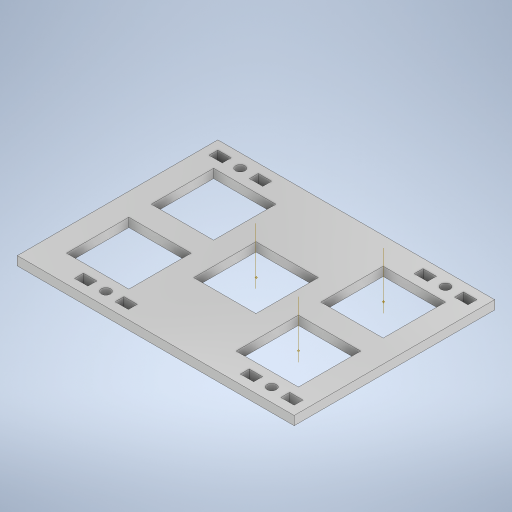
# Autodesk Inventor part: tc_base_plate
Saved by Autodesk Inventor 2024.1 (Build 281209000, 209)
## iProperties
Created: 2019-07-03
Part Number: tc_base_plate
Material: Acier inoxydable
Document SubType Name: Modeling
Designer: Thibault
Density: 8 g/cm^3
Appearance: Aluminium - Poli
Mass: 33.3223 g
Surface Area: 56.2435 cm^2
Volume: 4.16528 cm^3
tc_base_width: 62,200 mm
tc_base_support_dist: 37,050 mm
Author: Thibault
Autodesk Inventor part; units mm, degrees
ref_plane "YZ Plane" through (0, 0, 0) normal (1, 0, 0) x (0, 1, 0)
ref_plane "XZ Plane" through (0, 0, 0) normal (0, 1, 0) x (-1, 0, 0)
ref_plane "XY Plane" through (0, 0, 0) normal (0, 0, 1) x (1, 0, 0)
sketch "anchor" plane through (0, 0, 0) normal (0, 0, 1) x (1, 0, 0)
  circle A0 centre (94.2814, 48.5827) radius 0.85
  line L0 (91.2814, 49.5827) -> (87.2814, 49.5827)
  line L1 (87.2814, 49.5827) -> (87.2814, 47.5827)
  line L2 (87.2814, 47.5827) -> (91.2814, 47.5827)
  line L3 (91.2814, 47.5827) -> (91.2814, 49.5827)
  line L4 (101.2814, 49.5827) -> (97.2814, 49.5827)
  line L5 (97.2814, 49.5827) -> (97.2814, 47.5827)
  line L6 (97.2814, 47.5827) -> (101.2814, 47.5827)
  line L7 (101.2814, 47.5827) -> (101.2814, 49.5827)
  line L8 (91.2814, 49.5827) -> (97.2814, 47.5827) construction
  line L9 (97.2814, 49.5827) -> (91.2814, 47.5827) construction
  line L10 (87.2814, 51.1827) -> (101.2814, 51.1827)
  point P0 (103.5798, 50.1132)
  point P1 (94.2814, 48.5827)
  dimension "d226" = 1.7
  dimension "d230" = 4
  dimension "d231" = 2
  dimension "d237" = 4
  dimension "d245" = 1.6
  dimension "d247" = 6
  measures "d226" diameter of A0
  measures "d230" distance of L2.end L1.end
  measures "d231" distance of L1.end L0.end
  measures "d237" distance of L6.end L5.end
  measures "d245" distance between parallel lines of L0 L10
  measures "d247" distance between parallel lines of L5 L3
sketch "screw_anchor" plane through (0, 0, 0) normal (0, 0, 1) x (1, 0, 0)
  point P0 (61.1245, 15.5217)
  dimension "d155" = 14
  dimension "d156" = 19.05
  dimension "d157" = 19.05
  dimension "d158" = 19.05
  dimension "d159" = 28.575
  dimension "d160" = 19.05
  dimension "d161" = 2
  dimension "d162" = 2
  dimension "d163" = 2
  dimension "d164" = 2
  dimension "d165" = 2
  dimension "d166" = 1
  dimension "d167" = 5
  dimension "d168" = 5
  dimension "d169" = 4
sketch "Anchor (nut side)" plane through (0, 0, 0) normal (0, 0, 1) x (1, 0, 0)
  line L0 (11.1, 0) -> (9.1, 0)
  line L1 (9.1, 0) -> (9.1, -2)
  line L2 (9.1, -2) -> (9.9, -2)
  line L3 (9.9, -2) -> (9.9, -4)
  line L4 (6.2, -4) -> (6.2, -2)
  line L5 (6.2, -2) -> (7, -2)
  line L6 (7, -2) -> (7, 0)
  line L7 (7, 0) -> (5, 0)
  line L8 (2, 0) -> (2, 2)
  line L9 (2, 0) -> (3, 0) construction
  line L10 (2, 2) -> (5, 2)
  line L11 (5, 2) -> (5, 0)
  line L12 (11.1, 0) -> (11.1, 2)
  line L13 (11.1, 2) -> (14.1, 2)
  line L14 (14.1, 2) -> (14.1, 0)
  line L15 (0, 0) -> (2, 0)
  line L16 (14.1, 0) -> (16.1, 0)
  line L17 (6.2, -4) -> (7, -4)
  line L18 (9.9, -4) -> (9.1, -4)
  line L19 (7, -4) -> (7, -6.25)
  line L20 (9.1, -4) -> (9.1, -6.25)
  line L21 (7.25, -6.5) -> (8.05, -6.5)
  arc A0 (7, -6.25) -> (7.25, -6.5) centre (7.25, -6.25) ccw
  arc A1 (8.85, -6.5) -> (9.1, -6.25) centre (8.85, -6.25) ccw
  line L22 (8.05, -6.5) -> (8.85, -6.5)
  line L23 (8.05, -3.8983) -> (8.05, -9.959) construction
  point P0 (9.1321, -0.6227)
  point P1 (7, -6.5)
  point P2 (9.1, -6.5)
  dimension "d3" = 2
  dimension "d7" = 6.1
  dimension "d10" = 2
  dimension "d11" = 2
  dimension "d12" = 0.8
  dimension "d13" = 2
  dimension "d14" = 0.8
  dimension "d15" = 2.1
  dimension "d18" = 2
  dimension "d19" = 0.8
  dimension "d20" = 0.8
  dimension "d21" = 2.5
  dimension "d22" = 2.5
  dimension "d23" = 2.1
  dimension "d38" = 2
  dimension "d39" = 0.25
  dimension "d120" = 3
  measures "d3" distance of L15.start L8.start
  measures "d7" distance of L7.end L0.start
  measures "d10" distance of L0.start L0.end
  measures "d11" distance of L0.end L1.end
  measures "d12" distance of L1.end L2.end
  measures "d13" distance of L2.end L3.end
  measures "d14" distance of L4.end L5.end
  measures "d15" distance of L6.end L0.end
  measures "d18" distance of L14.end L16.end
  measures "d19" distance of L4.start L17.end
  measures "d20" distance of L3.end L18.end
  measures "d21" distance of L17.end point (7, -6.5)
  measures "d22" distance of L18.end point (9.1, -6.5)
  measures "d23" distance of L17.end L18.end
  measures "d38" distance between parallel lines of L15 L10
  measures "d39" radius of A0
  measures "d120" distance of L8.end L10.end
sketch "Anchor (screw side)" plane through (0, 0, 0) normal (0, 0, 1) x (1, 0, 0)
  circle A0 centre (93.8994, 50.2542) radius 1.05
  line L0 (90.8494, 51.2542) -> (87.8494, 51.2542)
  line L1 (87.8494, 51.2542) -> (87.8494, 49.2542)
  line L2 (87.8494, 49.2542) -> (90.8494, 49.2542)
  line L3 (90.8494, 49.2542) -> (90.8494, 51.2542)
  line L4 (99.9494, 51.2542) -> (96.9494, 51.2542)
  line L5 (96.9494, 51.2542) -> (96.9494, 49.2542)
  line L6 (96.9494, 49.2542) -> (99.9494, 49.2542)
  line L7 (99.9494, 49.2542) -> (99.9494, 51.2542)
  line L8 (90.8494, 51.2542) -> (96.9494, 49.2542) construction
  line L9 (96.9494, 51.2542) -> (90.8494, 49.2542) construction
  line L10 (85.8494, 53.2542) -> (101.9494, 53.2542) construction
  line L11 (101.9494, 53.2542) -> (101.9494, 47.2542) construction
  line L12 (101.9494, 47.2542) -> (85.8494, 47.2542) construction
  line L13 (85.8494, 47.2542) -> (85.8494, 53.2542) construction
  point P0 (103.5798, 50.1132)
  dimension "d27" = 2.1
  dimension "d28" = 3
  dimension "d29" = 2
  dimension "slot_distance" = 6.1
  dimension "d34" = 2
  dimension "d35" = 2
  dimension "d36" = 2
  dimension "d37" = 2
  measures "d27" diameter of A0
  measures "d28" distance of L2.end L1.end
  measures "d29" distance of L1.end L0.end
  measures "slot_distance" distance between parallel lines of L5 L3
  measures "d34" distance between parallel lines of L0 L10
  measures "d35" distance between parallel lines of L12 L2
  measures "d36" distance between parallel lines of L11 L7
  measures "d37" distance between parallel lines of L13 L1
sketch "Screwless anchor (male)" plane through (0, 0, 0) normal (0, 0, 1) x (1, 0, 0)
  line L0 (2, 0) -> (2, 2)
  line L1 (2, 0) -> (3, 0) construction
  line L2 (2, 2) -> (5, 2)
  line L3 (5, 2) -> (5, 0)
  line L4 (11.1, 0) -> (11.1, 2)
  line L5 (11.1, 2) -> (14.1, 2)
  line L6 (14.1, 2) -> (14.1, 0)
  line L7 (0, 0) -> (2, 0)
  line L8 (14.1, 0) -> (16.1, 0)
  line L9 (5, 0) -> (11.1, 0)
  point P0 (9.1321, -0.6227)
  dimension "d81" = 2
  dimension "d83" = 6.1
  dimension "d92" = 2
  dimension "d100" = 2
  dimension "d119" = 3
  measures "d81" distance of L7.start L0.start
  measures "d83" distance of L3.end L4.start
  measures "d92" distance of L6.end L8.end
  measures "d100" distance between parallel lines of L7 L2
  measures "d119" distance of L0.end L2.end
sketch "Screwless anchor (female)" plane through (0, 0, 0) normal (0, 0, 1) x (1, 0, 0)
  line L0 (91.6814, 51.6592) -> (88.6814, 51.6592)
  line L1 (88.6814, 51.6592) -> (88.6814, 49.6592)
  line L2 (88.6814, 49.6592) -> (91.6814, 49.6592)
  line L3 (91.6814, 49.6592) -> (91.6814, 51.6592)
  line L4 (100.7814, 51.6592) -> (97.7814, 51.6592)
  line L5 (97.7814, 51.6592) -> (97.7814, 49.6592)
  line L6 (97.7814, 49.6592) -> (100.7814, 49.6592)
  line L7 (100.7814, 49.6592) -> (100.7814, 51.6592)
  line L8 (86.6814, 53.6592) -> (102.7814, 53.6592) construction
  line L9 (102.7814, 53.6592) -> (102.7814, 47.6592) construction
  line L10 (102.7814, 47.6592) -> (86.6814, 47.6592) construction
  line L11 (86.6814, 47.6592) -> (86.6814, 53.6592) construction
  point P0 (103.5798, 50.1132)
  dimension "d106" = 3
  dimension "d107" = 2
  dimension "d108_1" = 3
  dimension "d109_1" = 6.1
  dimension "d110_1" = 2
  dimension "d111" = 2
  dimension "d112" = 2
  dimension "d113" = 2
  measures "d106" distance of L2.end L1.end
  measures "d107" distance of L1.end L0.end
  measures "d108_1" distance of L6.end L5.end
  measures "d109_1" distance between parallel lines of L5 L3
  measures "d110_1" distance between parallel lines of L0 L8
  measures "d111" distance between parallel lines of L10 L2
  measures "d112" distance between parallel lines of L9 L7
  measures "d113" distance between parallel lines of L11 L1
sketch "Esquisse2" plane through (0, 0, 0) normal (0, 1, 0) x (-1, 0, 0)
  line L0 (15.3814, -6.8116) -> (1.3814, -6.8116)
  line L1 (1.3814, -6.8116) -> (1.3814, 7.1884)
  line L2 (1.3814, 7.1884) -> (15.3814, 7.1884)
  line L3 (15.3814, 7.1884) -> (15.3814, -6.8116)
  line L4 (15.3814, -25.8616) -> (1.3814, -25.8616)
  line L5 (1.3814, -25.8616) -> (1.3814, -11.8616)
  line L6 (1.3814, -11.8616) -> (15.3814, -11.8616)
  line L7 (15.3814, -11.8616) -> (15.3814, -25.8616)
  line L8 (34.4314, -16.3366) -> (20.4314, -16.3366)
  line L9 (20.4314, -16.3366) -> (20.4314, -2.3366)
  line L10 (20.4314, -2.3366) -> (34.4314, -2.3366)
  line L11 (34.4314, -2.3366) -> (34.4314, -16.3366)
  line L12 (58.5314, -31.8616) -> (-3.6686, -31.8616)
  line L13 (-3.6686, -31.8616) -> (-3.6686, 13.1884)
  line L14 (58.5314, -31.8616) -> (58.5314, 13.1884)
  line L15 (58.5314, 13.1884) -> (-3.6686, 13.1884)
  line L16 (53.4814, -25.8616) -> (39.4814, -25.8616)
  line L17 (39.4814, -25.8616) -> (39.4814, -11.8616)
  line L18 (39.4814, -11.8616) -> (53.4814, -11.8616)
  line L19 (53.4814, -11.8616) -> (53.4814, -25.8616)
  line L20 (53.4814, -6.8116) -> (39.4814, -6.8116)
  line L21 (39.4814, -6.8116) -> (39.4814, 7.1884)
  line L22 (39.4814, 7.1884) -> (53.4814, 7.1884)
  line L23 (53.4814, 7.1884) -> (53.4814, -6.8116)
  circle A0 centre (41.622, 10.1884) radius 1.05
  line L24 (38.572, 11.1884) -> (35.572, 11.1884)
  line L25 (35.572, 11.1884) -> (35.572, 9.1884)
  line L26 (35.572, 9.1884) -> (38.572, 9.1884)
  line L27 (38.572, 9.1884) -> (38.572, 11.1884)
  line L28 (47.672, 11.1884) -> (44.672, 11.1884)
  line L29 (44.672, 11.1884) -> (44.672, 9.1884)
  line L30 (44.672, 9.1884) -> (47.672, 9.1884)
  line L31 (47.672, 9.1884) -> (47.672, 11.1884)
  line L32 (38.572, 11.1884) -> (44.672, 9.1884) construction
  line L33 (44.672, 11.1884) -> (38.572, 9.1884) construction
  line L34 (33.572, 13.1884) -> (49.672, 13.1884) construction
  line L35 (49.672, 13.1884) -> (49.672, 7.1884) construction
  line L36 (49.672, 7.1884) -> (33.572, 7.1884) construction
  line L37 (33.572, 7.1884) -> (33.572, 13.1884) construction
  circle A1 centre (4.3814, 10.1884) radius 1.05
  line L38 (1.3314, 11.1884) -> (-1.6686, 11.1884)
  line L39 (-1.6686, 11.1884) -> (-1.6686, 9.1884)
  line L40 (-1.6686, 9.1884) -> (1.3314, 9.1884)
  line L41 (1.3314, 9.1884) -> (1.3314, 11.1884)
  line L42 (10.4314, 11.1884) -> (7.4314, 11.1884)
  line L43 (7.4314, 11.1884) -> (7.4314, 9.1884)
  line L44 (7.4314, 9.1884) -> (10.4314, 9.1884)
  line L45 (10.4314, 9.1884) -> (10.4314, 11.1884)
  line L46 (1.3314, 11.1884) -> (7.4314, 9.1884) construction
  line L47 (7.4314, 11.1884) -> (1.3314, 9.1884) construction
  line L48 (-3.6686, 13.1884) -> (12.4314, 13.1884) construction
  line L49 (12.4314, 13.1884) -> (12.4314, 7.1884) construction
  line L50 (12.4314, 7.1884) -> (-3.6686, 7.1884) construction
  line L51 (-3.6686, 7.1884) -> (-3.6686, 13.1884) construction
  circle A2 centre (4.3814, -28.8616) radius 1.05
  line L52 (1.3314, -27.8616) -> (-1.6686, -27.8616)
  line L53 (-1.6686, -27.8616) -> (-1.6686, -29.8616)
  line L54 (-1.6686, -29.8616) -> (1.3314, -29.8616)
  line L55 (1.3314, -29.8616) -> (1.3314, -27.8616)
  line L56 (10.4314, -27.8616) -> (7.4314, -27.8616)
  line L57 (7.4314, -27.8616) -> (7.4314, -29.8616)
  line L58 (7.4314, -29.8616) -> (10.4314, -29.8616)
  line L59 (10.4314, -29.8616) -> (10.4314, -27.8616)
  line L60 (1.3314, -27.8616) -> (7.4314, -29.8616) construction
  line L61 (7.4314, -27.8616) -> (1.3314, -29.8616) construction
  line L62 (-3.6686, -25.8616) -> (12.4314, -25.8616) construction
  line L63 (12.4314, -25.8616) -> (12.4314, -31.8616) construction
  line L64 (12.4314, -31.8616) -> (-3.6686, -31.8616) construction
  line L65 (-3.6686, -31.8616) -> (-3.6686, -25.8616) construction
  circle A3 centre (50.4814, -28.8616) radius 1.05
  line L66 (47.4314, -27.8616) -> (44.4314, -27.8616)
  line L67 (44.4314, -27.8616) -> (44.4314, -29.8616)
  line L68 (44.4314, -29.8616) -> (47.4314, -29.8616)
  line L69 (47.4314, -29.8616) -> (47.4314, -27.8616)
  line L70 (56.5314, -27.8616) -> (53.5314, -27.8616)
  line L71 (53.5314, -27.8616) -> (53.5314, -29.8616)
  line L72 (53.5314, -29.8616) -> (56.5314, -29.8616)
  line L73 (56.5314, -29.8616) -> (56.5314, -27.8616)
  line L74 (47.4314, -27.8616) -> (53.5314, -29.8616) construction
  line L75 (53.5314, -27.8616) -> (47.4314, -29.8616) construction
  line L76 (42.4314, -25.8616) -> (58.5314, -25.8616) construction
  line L77 (58.5314, -25.8616) -> (58.5314, -31.8616) construction
  line L78 (58.5314, -31.8616) -> (42.4314, -31.8616) construction
  line L79 (42.4314, -31.8616) -> (42.4314, -25.8616) construction
  point P0 (38.4348, -22.3397)
  point P1 (39.3203, -53.3777)
  point P2 (34.5306, -31.8616)
  point P3 (1.2703, -53.3777)
  point P4 (20.4314, -9.3366)
  dimension "tc_base_support_dist" = 37.05
  dimension "d108" = 14
  dimension "d110" = 19.05
  dimension "d260" = 2
  dimension "d276" = 14
  dimension "d277" = 14
  dimension "d278" = 19.05
  dimension "d279" = 14
  dimension "d280" = 14
  dimension "d282" = 19.05
  dimension "d283" = 9.525
  dimension "d284" = 9.525
  dimension "d285" = 14
  dimension "d286" = 19.05
  dimension "d287" = 14
  dimension "d288" = 19.05
  dimension "d289" = 19.05
  constraints: 48 end point, 11 horizontal, 10 parallel, 8 perpendicular, 5 vertical, 3 collinear, 1 midpoint, 1 point on line
  measures "d108" distance of L1.end L2.end
  measures "d110" distance of L0.end L4.end
  measures "d276" distance of L17.end L18.end
  measures "d277" distance of L16.end L17.end
  measures "d278" distance from line of point (20.431, -9.337) L17
  measures "d279" distance of L21.end L22.end
  measures "d280" distance of L20.end L21.end
  measures "d282" distance between parallel lines of L9 L21
  measures "d285" distance of L8.start L8.end
  measures "d286" distance between parallel lines of L7 L11
  measures "d287" distance of L6.end L4.start
  measures "d288" distance between parallel lines of L17 L14
  measures "d289" distance between parallel lines of L7 L13
extrude "Base" add sketch "Esquisse2" along normal blind 2
derived "shared_parameters.ipt"
